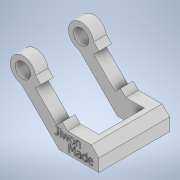
# Autodesk Inventor part: 10-1
Saved by Autodesk Inventor 2022 (Build 260153000, 153)
## iProperties
Created: 2021-09-12
Part Number: 10-1
Material: 일반
Document SubType Name: Modeling
Designer: 서울공업고등학교
Density: 1 g/cm^3
Appearance: 기본값
Author: 서울공업고등학교
Autodesk Inventor part; units mm, degrees
ref_plane "YZ Plane" through (0, 0, 0) normal (1, 0, 0) x (0, 1, 0)
ref_plane "XZ Plane" through (0, 0, 0) normal (0, 1, 0) x (-1, 0, 0)
ref_plane "XY Plane" through (0, 0, 0) normal (0, 0, 1) x (1, 0, 0)
sketch "스케치1" plane through (0, 0, 0) normal (0, 0, 1) x (1, 0, 0)
  circle A0 centre (0, 0) radius 3
  circle A1 centre (0, 0) radius 5
  line L0 (-0.7071, -4.9497) -> (14.3431, -20)
  line L1 (14.3431, -20) -> (30, -20)
  line L2 (30, -20) -> (30, -12)
  line L3 (30, -12) -> (17.6569, -12)
  line L4 (17.6569, -12) -> (15.5563, -9.8995)
  line L5 (15.5563, -9.8995) -> (13.435, -12.0208)
  line L6 (13.435, -12.0208) -> (4.9497, -3.5355)
  line L7 (4.9497, -3.5355) -> (7.0711, -1.4142)
  line L8 (7.0711, -1.4142) -> (4.9497, 0.7071)
  line L9 (0, 0) -> (7.8579, -7.8579)
  dimension "d0" = 6
  dimension "d1" = 10
  dimension "d2" = 8
  dimension "d3" = 3
  dimension "d4" = 20
  dimension "d5" = 5
  dimension "d6" = 6
  dimension "d7" = 12
  dimension "d8" = 45
  dimension "d9" = 8
  dimension "d10" = 30
  dimension "d11" = 8
  constraints: 20 end point, 6 perpendicular, 2 centre point, 2 coincident, 2 parallel, 2 point on circle, 1 horizontal
  measures "d0" diameter of A0
  measures "d1" diameter of A1
  measures "d2" distance between parallel lines of L1 L3
  measures "d3" distance between parallel lines of L6 L8
  measures "d4" distance from line of L1 point (0, 0)
  measures "d5" distance between parallel lines of L0 L6
  measures "d6" distance from line of L7 point (0, 0)
  measures "d7" distance between parallel lines of L5 L7
  measures "d8" angle of L1 L0
  measures "d9" distance between parallel lines of L0 L4
  measures "d10" horizontal distance of L1.end point (0, 0)
  measures "d11" diameter of L0 L9
extrude "돌출1" add sketch "스케치1" along normal mid plane 28
sketch "스케치2" plane through (0, 0, 0) normal (0, 0, 1) x (1, 0, 0)
  line L0 (-7.8, 7.5225) -> (25, 7.5225)
  line L1 (25, 7.5225) -> (25, -21.6426)
  line L2 (25, -21.6426) -> (-7.8, -21.6426)
  line L3 (-7.8, -21.6426) -> (-7.8, 7.5225)
  line L4 (30, -20) -> (30, -12) projected
  point P0 (0, 0)
  dimension "d14" = 5
  constraints: 8 end point, 2 parallel, 1 horizontal, 1 perpendicular
  measures "d14" distance between parallel lines of L1 L4
extrude "돌출2" cut sketch "스케치2" along normal mid plane 18
chamfer "모따기1" distance 3 angle 45 1 edges at (30, -12, 0)
sketch "스케치3" plane through (0, 0, 14) normal (0, 0, 1) x (1, 0, 0)
  line L0 (12.6192, -12.4113) -> (34.3084, -12.4113) construction
  line L1 (34.3084, -12.4113) -> (34.3084, -15.6594) construction
  line L2 (34.3084, -15.6594) -> (12.6192, -15.6594) construction
  line L3 (12.6192, -15.6594) -> (12.6192, -12.4113) construction
  spline S0 degree 2 poles (14.0765, -14.6862) (14.0765, -15.0864) (13.5874, -15.5211) (13.1749, -15.5211) knots 0 0 0 1 2 2 2
  spline S1 degree 2 poles (13.1749, -15.5211) (13.0761, -15.5211) (12.7476, -15.4865) (12.6365, -15.4618) knots 0 0 0 1 2 2 2
  line L4 (12.6365, -15.4618) -> (12.6365, -15.0715)
  line L5 (12.6365, -15.0715) -> (12.6587, -15.0715)
  spline S2 degree 2 poles (12.6587, -15.0715) (12.7427, -15.1012) (12.9922, -15.1704) (13.1206, -15.1704) knots 0 0 0 1 2 2 2
  spline S3 degree 2 poles (13.1206, -15.1704) (13.3083, -15.1704) (13.5331, -15.0839) (13.585, -15.0049) knots 0 0 0 1 2 2 2
  spline S4 degree 2 poles (13.585, -15.0049) (13.6418, -14.9233) (13.6714, -14.6862) (13.6714, -14.5306) knots 0 0 0 1 2 2 2
  line L6 (13.6714, -14.5306) -> (13.6714, -12.7547)
  line L7 (13.6714, -12.7547) -> (13.0267, -12.7547)
  line L8 (13.0267, -12.7547) -> (13.0267, -12.4311)
  line L9 (13.0267, -12.4311) -> (14.0765, -12.4311)
  line L10 (14.0765, -12.4311) -> (14.0765, -14.6862)
  line L11 (15.0373, -15.4791) -> (14.652, -15.4791)
  line L12 (14.652, -15.4791) -> (14.652, -13.1919)
  line L13 (14.652, -13.1919) -> (15.0373, -13.1919)
  line L14 (15.0373, -13.1919) -> (15.0373, -15.4791)
  line L15 (15.0645, -12.8115) -> (14.6273, -12.8115)
  line L16 (14.6273, -12.8115) -> (14.6273, -12.4113)
  line L17 (14.6273, -12.4113) -> (15.0645, -12.4113)
  line L18 (15.0645, -12.4113) -> (15.0645, -12.8115)
  line L19 (18.3743, -13.1919) -> (17.7939, -15.4791)
  line L20 (17.7939, -15.4791) -> (17.4382, -15.4791)
  line L21 (17.4382, -15.4791) -> (16.88, -13.7155)
  line L22 (16.88, -13.7155) -> (16.3242, -15.4791)
  line L23 (16.3242, -15.4791) -> (15.971, -15.4791)
  line L24 (15.971, -15.4791) -> (15.3856, -13.1919)
  line L25 (15.3856, -13.1919) -> (15.7857, -13.1919)
  line L26 (15.7857, -13.1919) -> (16.1908, -14.9629)
  line L27 (16.1908, -14.9629) -> (16.7318, -13.1919)
  line L28 (16.7318, -13.1919) -> (17.0504, -13.1919)
  line L29 (17.0504, -13.1919) -> (17.6061, -14.9629)
  line L30 (17.6061, -14.9629) -> (17.9865, -13.1919)
  line L31 (17.9865, -13.1919) -> (18.3743, -13.1919)
  spline S5 degree 2 poles (20.5924, -14.3355) (20.5924, -14.9135) (20.0366, -15.5433) (19.5723, -15.5433) knots 0 0 0 1 2 2 2
  spline S6 degree 2 poles (19.5723, -15.5433) (19.0956, -15.5433) (18.5497, -14.8937) (18.5497, -14.3355) knots 0 0 0 1 2 2 2
  spline S7 degree 2 poles (18.5497, -14.3355) (18.5497, -13.7624) (19.1129, -13.1276) (19.5723, -13.1276) knots 0 0 0 1 2 2 2
  spline S8 degree 2 poles (19.5723, -13.1276) (20.0366, -13.1276) (20.5924, -13.76) (20.5924, -14.3355) knots 0 0 0 1 2 2 2
  spline S9 degree 2 poles (20.1947, -14.3355) (20.1947, -13.8909) (19.8712, -13.4586) (19.5723, -13.4586) knots 0 0 0 1 2 2 2
  spline S10 degree 2 poles (19.5723, -13.4586) (19.2734, -13.4586) (18.9474, -13.8909) (18.9474, -14.3355) knots 0 0 0 1 2 2 2
  spline S11 degree 2 poles (18.9474, -14.3355) (18.9474, -14.7677) (19.2734, -15.2123) (19.5723, -15.2123) knots 0 0 0 1 2 2 2
  spline S12 degree 2 poles (19.5723, -15.2123) (19.8687, -15.2123) (20.1947, -14.7751) (20.1947, -14.3355) knots 0 0 0 1 2 2 2
  line L32 (22.7833, -15.4791) -> (22.398, -15.4791)
  line L33 (22.398, -15.4791) -> (22.398, -14.1749)
  spline S13 degree 2 poles (22.398, -14.1749) (22.398, -14.0169) (22.3683, -13.7452) (22.3239, -13.6636) knots 0 0 0 1 2 2 2
  spline S14 degree 2 poles (22.3239, -13.6636) (22.277, -13.5772) (22.109, -13.4932) (21.9657, -13.4932) knots 0 0 0 1 2 2 2
  spline S15 degree 2 poles (21.9657, -13.4932) (21.8225, -13.4932) (21.5187, -13.6464) (21.3729, -13.7699) knots 0 0 0 1 2 2 2
  line L34 (21.3729, -13.7699) -> (21.3729, -15.4791)
  line L35 (21.3729, -15.4791) -> (20.9876, -15.4791)
  line L36 (20.9876, -15.4791) -> (20.9876, -13.1919)
  line L37 (20.9876, -13.1919) -> (21.3729, -13.1919)
  line L38 (21.3729, -13.1919) -> (21.3729, -13.4463)
  spline S16 degree 2 poles (21.3729, -13.4463) (21.5458, -13.2907) (21.8793, -13.1276) (22.067, -13.1276) knots 0 0 0 1 2 2 2
  spline S17 degree 2 poles (22.067, -13.1276) (22.4029, -13.1276) (22.7833, -13.5722) (22.7833, -13.9946) knots 0 0 0 1 2 2 2
  line L39 (22.7833, -13.9946) -> (22.7833, -15.4791)
  line L40 (20.7777, -18.9791) -> (20.3726, -18.9791)
  line L41 (20.3726, -18.9791) -> (20.3726, -16.3535)
  line L42 (20.3726, -16.3535) -> (19.5772, -18.1393)
  line L43 (19.5772, -18.1393) -> (19.3302, -18.1393)
  line L44 (19.3302, -18.1393) -> (18.5423, -16.3535)
  line L45 (18.5423, -16.3535) -> (18.5423, -18.9791)
  line L46 (18.5423, -18.9791) -> (18.1644, -18.9791)
  line L47 (18.1644, -18.9791) -> (18.1644, -15.9311)
  line L48 (18.1644, -15.9311) -> (18.7177, -15.9311)
  line L49 (18.7177, -15.9311) -> (19.4784, -17.628)
  line L50 (19.4784, -17.628) -> (20.2145, -15.9311)
  line L51 (20.2145, -15.9311) -> (20.7777, -15.9311)
  line L52 (20.7777, -15.9311) -> (20.7777, -18.9791)
  spline S18 degree 2 poles (22.64, -18.737) (22.5931, -18.7716) (22.435, -18.8951) (22.3609, -18.9322) knots 0 0 0 1 2 2 2
  spline S19 degree 2 poles (22.3609, -18.9322) (22.2597, -18.9865) (22.0695, -19.0433) (21.8966, -19.0433) knots 0 0 0 1 2 2 2
  spline S20 degree 2 poles (21.8966, -19.0433) (21.7558, -19.0433) (21.5014, -18.9371) (21.405, -18.8408) knots 0 0 0 1 2 2 2
  spline S21 degree 2 poles (21.405, -18.8408) (21.3136, -18.7469) (21.2025, -18.4703) (21.2025, -18.3171) knots 0 0 0 1 2 2 2
  spline S22 degree 2 poles (21.2025, -18.3171) (21.2025, -18.08) (21.4026, -17.7441) (21.6199, -17.6478) knots 0 0 0 1 2 2 2
  spline S23 degree 2 poles (21.6199, -17.6478) (21.8126, -17.5588) (22.3362, -17.4922) (22.64, -17.4749) knots 0 0 0 1 2 2 2
  line L53 (22.64, -17.4749) -> (22.64, -17.4008)
  spline S24 degree 2 poles (22.64, -17.4008) (22.64, -17.2674) (22.5585, -17.1019) (22.4844, -17.055) knots 0 0 0 1 2 2 2
  spline S25 degree 2 poles (22.4844, -17.055) (22.4103, -17.008) (22.1979, -16.9784) (22.0843, -16.9784) knots 0 0 0 1 2 2 2
  spline S26 degree 2 poles (22.0843, -16.9784) (21.9509, -16.9784) (21.5903, -17.0574) (21.41, -17.134) knots 0 0 0 1 2 2 2
  line L54 (21.41, -17.134) -> (21.3877, -17.134)
  line L55 (21.3877, -17.134) -> (21.3877, -16.7413)
  spline S27 degree 2 poles (21.3877, -16.7413) (21.494, -16.7116) (21.8916, -16.6375) (22.0868, -16.6375) knots 0 0 0 1 2 2 2
  spline S28 degree 2 poles (22.0868, -16.6375) (22.3239, -16.6375) (22.6475, -16.7116) (22.7759, -16.808) knots 0 0 0 1 2 2 2
  spline S29 degree 2 poles (22.7759, -16.808) (22.9019, -16.9018) (23.0254, -17.2007) (23.0254, -17.4156) knots 0 0 0 1 2 2 2
  line L56 (23.0254, -17.4156) -> (23.0254, -18.9791)
  line L57 (23.0254, -18.9791) -> (22.64, -18.9791)
  line L58 (22.64, -18.9791) -> (22.64, -18.737)
  line L59 (22.64, -18.4159) -> (22.64, -17.7811)
  spline S30 degree 2 poles (22.64, -17.7811) (22.5017, -17.7935) (22.0843, -17.8355) (21.9534, -17.875) knots 0 0 0 1 2 2 2
  spline S31 degree 2 poles (21.9534, -17.875) (21.8002, -17.9219) (21.6002, -18.1171) (21.6002, -18.29) knots 0 0 0 1 2 2 2
  spline S32 degree 2 poles (21.6002, -18.29) (21.6002, -18.4876) (21.8225, -18.6876) (22.0349, -18.6876) knots 0 0 0 1 2 2 2
  spline S33 degree 2 poles (22.0349, -18.6876) (22.2152, -18.6876) (22.5116, -18.532) (22.64, -18.4159) knots 0 0 0 1 2 2 2
  line L60 (25.325, -18.9791) -> (24.9396, -18.9791)
  line L61 (24.9396, -18.9791) -> (24.9396, -18.7469)
  spline S34 degree 2 poles (24.9396, -18.7469) (24.8507, -18.821) (24.7198, -18.9198) (24.6309, -18.9618) knots 0 0 0 1 2 2 2
  spline S35 degree 2 poles (24.6309, -18.9618) (24.5494, -19.0013) (24.374, -19.0433) (24.2579, -19.0433) knots 0 0 0 1 2 2 2
  spline S36 degree 2 poles (24.2579, -19.0433) (24.0702, -19.0433) (23.754, -18.8877) (23.6429, -18.737) knots 0 0 0 1 2 2 2
  spline S37 degree 2 poles (23.6429, -18.737) (23.5317, -18.5864) (23.4082, -18.1418) (23.4082, -17.8528) knots 0 0 0 1 2 2 2
  spline S38 degree 2 poles (23.4082, -17.8528) (23.4082, -17.5514) (23.5638, -17.1118) (23.6997, -16.9463) knots 0 0 0 1 2 2 2
  spline S39 degree 2 poles (23.6997, -16.9463) (23.8257, -16.7981) (24.1789, -16.6276) (24.374, -16.6276) knots 0 0 0 1 2 2 2
  spline S40 degree 2 poles (24.374, -16.6276) (24.5444, -16.6276) (24.7988, -16.7042) (24.9396, -16.7833) knots 0 0 0 1 2 2 2
  line L62 (24.9396, -16.7833) -> (24.9396, -15.7953)
  line L63 (24.9396, -15.7953) -> (25.325, -15.7953)
  line L64 (25.325, -15.7953) -> (25.325, -18.9791)
  line L65 (24.9396, -18.4233) -> (24.9396, -17.1019)
  spline S41 degree 2 poles (24.9396, -17.1019) (24.7964, -17.0327) (24.5691, -16.9809) (24.4382, -16.9809) knots 0 0 0 1 2 2 2
  spline S42 degree 2 poles (24.4382, -16.9809) (24.1418, -16.9809) (23.8059, -17.4255) (23.8059, -17.8454) knots 0 0 0 1 2 2 2
  spline S43 degree 2 poles (23.8059, -17.8454) (23.8059, -18.2504) (24.0628, -18.6778) (24.3468, -18.6778) knots 0 0 0 1 2 2 2
  spline S44 degree 2 poles (24.3468, -18.6778) (24.4975, -18.6778) (24.8038, -18.5394) (24.9396, -18.4233) knots 0 0 0 1 2 2 2
  spline S45 degree 2 poles (26.8761, -19.031) (26.3278, -19.031) (25.7251, -18.4159) (25.7251, -17.8478) knots 0 0 0 1 2 2 2
  spline S46 degree 2 poles (25.7251, -17.8478) (25.7251, -17.2896) (26.3105, -16.6276) (26.7823, -16.6276) knots 0 0 0 1 2 2 2
  spline S47 degree 2 poles (26.7823, -16.6276) (26.9947, -16.6276) (27.3232, -16.7511) (27.4442, -16.8821) knots 0 0 0 1 2 2 2
  spline S48 degree 2 poles (27.4442, -16.8821) (27.5677, -17.013) (27.6986, -17.3909) (27.6986, -17.6651) knots 0 0 0 1 2 2 2
  line L66 (27.6986, -17.6651) -> (27.6986, -17.875)
  line L67 (27.6986, -17.875) -> (26.1154, -17.875)
  spline S49 degree 2 poles (26.1154, -17.875) (26.1154, -18.2727) (26.5155, -18.6951) (26.8712, -18.6951) knots 0 0 0 1 2 2 2
  spline S50 degree 2 poles (26.8712, -18.6951) (26.9972, -18.6951) (27.2417, -18.6382) (27.3405, -18.5938) knots 0 0 0 1 2 2 2
  spline S51 degree 2 poles (27.3405, -18.5938) (27.4442, -18.5444) (27.5875, -18.4579) (27.6344, -18.4184) knots 0 0 0 1 2 2 2
  line L68 (27.6344, -18.4184) -> (27.6566, -18.4184)
  line L69 (27.6566, -18.4184) -> (27.6566, -18.8383)
  spline S52 degree 2 poles (27.6566, -18.8383) (27.59, -18.8655) (27.3874, -18.9445) (27.3084, -18.9668) knots 0 0 0 1 2 2 2
  spline S53 degree 2 poles (27.3084, -18.9668) (27.1972, -18.9989) (27.0144, -19.031) (26.8761, -19.031) knots 0 0 0 1 2 2 2
  spline S54 degree 2 poles (27.3232, -17.5811) (27.3183, -17.4255) (27.254, -17.1982) (27.1923, -17.1216) knots 0 0 0 1 2 2 2
  spline S55 degree 2 poles (27.1923, -17.1216) (27.1256, -17.0352) (26.9156, -16.9438) (26.76, -16.9438) knots 0 0 0 1 2 2 2
  spline S56 degree 2 poles (26.76, -16.9438) (26.6069, -16.9438) (26.392, -17.0352) (26.3031, -17.1241) knots 0 0 0 1 2 2 2
  spline S57 degree 2 poles (26.3031, -17.1241) (26.2166, -17.2155) (26.1277, -17.4353) (26.1154, -17.5811) knots 0 0 0 1 2 2 2
  line L70 (26.1154, -17.5811) -> (27.3232, -17.5811)
  point P0 (0, 0)
  constraints: 2 other
extrude "돌출3" cut sketch "스케치3" against normal blind 1
